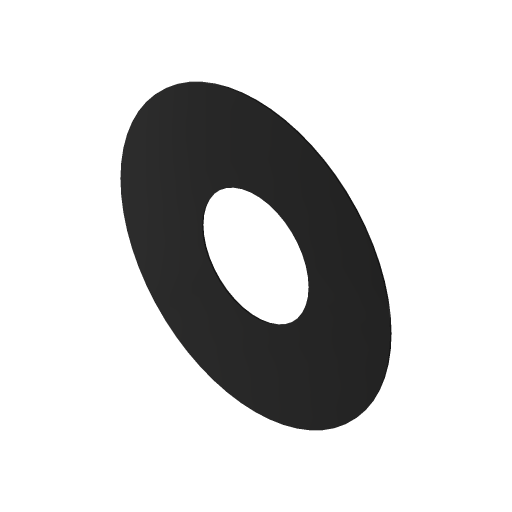
# Autodesk Inventor part: E-Stop Plate (Black)
Saved by Autodesk Inventor 2023.2 (Build 272271000, 271)
## iProperties
Created: 2021-03-05
Part Number: E-Stop Plate (Black)
Material: UHMW, Black
Document SubType Name: Modeling
Designer: Remo
Mass: 0.634081 g
Surface Area: 45.736 cm^2
Volume: 0.674554 cm^3
Density: 0.94 g/cm^3
Appearance: Smooth - Black
Author: Remo
Autodesk Inventor part; units mm, degrees
ref_plane "YZ Plane" through (0, 0, 0) normal (1, 0, 0) x (0, 1, 0)
ref_plane "XZ Plane" through (0, 0, 0) normal (0, 1, 0) x (-1, 0, 0)
ref_plane "XY Plane" through (0, 0, 0) normal (0, 0, 1) x (1, 0, 0)
sketch "Sketch1" plane through (0, 0, 0) normal (0, 0, 1) x (1, 0, 0)
  circle A0 centre (0, 0) radius 29.12 projected
  spline S0 degree 3 poles (-11.9075, -16.7717) (-12.086, -16.7855) (-12.2588, -16.8244) (-12.5934, -16.9566) (-12.7523, -17.0491) (-13.1401, -17.3576) (-13.3337, -17.6127) (-13.4879, -17.8856) knots -0.20259 -0.20259 -0.20259 -0.20259 -0.148567 -0.148567 -0.094046 -0.094046 0 0 0 0 projected
  spline S1 degree 3 poles (-10.0812, -17.2756) (-10.3794, -17.1072) (-10.7111, -16.9507) (-11.3404, -16.7781) (-11.626, -16.7509) (-11.9075, -16.7717) knots -0.178551 -0.178551 -0.178551 -0.178551 -0.084682 -0.084682 0 0 0 0 projected
  line L0 (-7.7154, -18.612) -> (-10.0812, -17.2756) projected
  line L1 (-11.1583, -24.7069) -> (-7.7154, -18.612) projected
  line L2 (-12.6894, -23.8419) -> (-11.1583, -24.7069) projected
  line L3 (-11.5622, -21.8466) -> (-12.6894, -23.8419) projected
  line L4 (-12.3624, -21.3946) -> (-11.5622, -21.8466) projected
  spline S2 degree 3 poles (-13.3296, -20.5811) (-13.2082, -20.736) (-13.0703, -20.8775) (-12.8431, -21.0755) (-12.6688, -21.2215) (-12.3624, -21.3946) knots -0.304465 -0.304465 -0.304465 -0.304465 -0.105593 -0.105593 0 0 0 0 projected
  spline S3 degree 3 poles (-13.7846, -19.6335) (-13.7433, -19.8022) (-13.685, -19.9651) (-13.5697, -20.2108) (-13.4849, -20.3798) (-13.3296, -20.5811) knots -0.211773 -0.211773 -0.211773 -0.211773 -0.07625 -0.07625 0 0 0 0 projected
  spline S4 degree 3 poles (-13.4879, -17.8856) (-13.5813, -18.0509) (-13.6584, -18.2235) (-13.7744, -18.5785) (-13.8153, -18.7636) (-13.8576, -19.177) (-13.845, -19.408) (-13.7846, -19.6335) knots -0.181189 -0.181189 -0.181189 -0.181189 -0.12469 -0.12469 -0.070002 -0.070002 0 0 0 0 projected
  spline S5 degree 3 poles (-3.098, -19.6093) (-3.5995, -19.53) (-4.1119, -19.5258) (-4.9872, -19.7428) (-5.336, -19.9081) (-5.8954, -20.327) (-6.2031, -20.6109) (-6.7632, -21.5612) (-6.9293, -22.1193) (-7.0183, -22.6822) knots -0.803042 -0.803042 -0.803042 -0.803042 -0.536977 -0.536977 -0.330685 -0.330685 -0.170955 -0.170955 0 0 0 0 projected
  spline S6 degree 3 poles (-0.3227, -23.741) (-0.2718, -23.4189) (-0.2455, -23.0908) (-0.2648, -22.4708) (-0.3034, -22.1789) (-0.5023, -21.4398) (-0.6961, -21.0977) (-1.1107, -20.5353) (-1.3922, -20.2811) (-2.1435, -19.8313) (-2.6154, -19.6856) (-3.098, -19.6093) knots -0.479254 -0.479254 -0.479254 -0.479254 -0.41452 -0.41452 -0.356105 -0.356105 -0.262594 -0.262594 -0.146589 -0.146589 0 0 0 0 projected
  spline S7 degree 3 poles (-4.2374, -26.8147) (-3.7386, -26.8936) (-3.2285, -26.8982) (-2.3601, -26.6833) (-2.015, -26.5203) (-1.4323, -26.0851) (-1.1292, -25.7911) (-0.5788, -24.861) (-0.4118, -24.3043) (-0.3227, -23.741) knots -0.728851 -0.728851 -0.728851 -0.728851 -0.500216 -0.500216 -0.324019 -0.324019 -0.171091 -0.171091 0 0 0 0 projected
  spline S8 degree 3 poles (-7.0183, -22.6822) (-7.0686, -23.0001) (-7.0951, -23.3241) (-7.079, -23.9356) (-7.043, -24.2235) (-6.8418, -24.9989) (-6.6342, -25.3416) (-6.2365, -25.8816) (-5.9526, -26.1383) (-5.1963, -26.5915) (-4.7225, -26.738) (-4.2374, -26.8147) knots -0.448983 -0.448983 -0.448983 -0.448983 -0.396063 -0.396063 -0.348437 -0.348437 -0.26439 -0.26439 -0.147326 -0.147326 0 0 0 0 projected
  spline S9 degree 3 poles (9.7964, -22.9748) (9.873, -23.1091) (9.9611, -23.2363) (10.1586, -23.4637) (10.2652, -23.5632) (10.5993, -23.8097) (10.8409, -23.9174) (11.3557, -24.0436) (11.7011, -24.0855) (12.6436, -23.9411) (13.1336, -23.7358) (13.5793, -23.4816) knots -0.573293 -0.573293 -0.573293 -0.573293 -0.495269 -0.495269 -0.421354 -0.421354 -0.285769 -0.285769 -0.153911 -0.153911 0 0 0 0 projected
  spline S10 degree 3 poles (10.1128, -20.6327) (9.9812, -20.7887) (9.8593, -20.9571) (9.6734, -21.2903) (9.6029, -21.4546) (9.5083, -21.8196) (9.4931, -22.0143) (9.5618, -22.4912) (9.6645, -22.7435) (9.7964, -22.9748) knots -0.267973 -0.267973 -0.267973 -0.267973 -0.2019 -0.2019 -0.14446 -0.14446 -0.079889 -0.079889 0 0 0 0 projected
  spline S11 degree 3 poles (11.1303, -19.6344) (10.9594, -19.7906) (10.7883, -19.9482) (10.4605, -20.2529) (10.3598, -20.3495) (10.1128, -20.6327) knots -0.233565 -0.233565 -0.233565 -0.233565 -0.112749 -0.112749 0 0 0 0 projected
  spline S12 degree 3 poles (11.5822, -18.5604) (11.612, -18.6128) (11.6358, -18.6685) (11.6628, -18.7815) (11.667, -18.8365) (11.6526, -18.9826) (11.6201, -19.0532) (11.5167, -19.2467) (11.3517, -19.4308) (11.1303, -19.6344) knots -0.147436 -0.147436 -0.147436 -0.147436 -0.130795 -0.130795 -0.115368 -0.115368 -0.09026 -0.09026 0 0 0 0 projected
  spline S13 degree 3 poles (10.9597, -18.282) (11.0119, -18.2769) (11.064, -18.2773) (11.169, -18.2893) (11.2208, -18.301) (11.3587, -18.3464) (11.4141, -18.3806) (11.5054, -18.451) (11.5486, -18.5016) (11.5822, -18.5604) knots -0.050985 -0.050985 -0.050985 -0.050985 -0.042849 -0.042849 -0.034581 -0.034581 -0.020323 -0.020323 0 0 0 0 projected
  spline S14 degree 3 poles (10.1862, -18.5403) (10.305, -18.4726) (10.4335, -18.4094) (10.6285, -18.342) (10.7569, -18.3024) (10.9597, -18.282) knots -0.181503 -0.181503 -0.181503 -0.181503 -0.061137 -0.061137 0 0 0 0 projected
  spline S15 degree 3 poles (8.7516, -20.2728) (8.8988, -19.8634) (9.1304, -19.5268) (9.5456, -18.9963) (9.8398, -18.7379) (10.1862, -18.5403) knots -0.202104 -0.202104 -0.202104 -0.202104 -0.119641 -0.119641 0 0 0 0 projected
  line L5 (8.6186, -20.3487) -> (8.7516, -20.2728) projected
  line L6 (7.826, -18.9592) -> (8.6186, -20.3487) projected
  spline S16 degree 3 poles (9.6327, -17.3866) (9.2693, -17.594) (8.9309, -17.8365) (8.3425, -18.3546) (8.0628, -18.6388) (7.826, -18.9592) knots -0.256315 -0.256315 -0.256315 -0.256315 -0.119514 -0.119514 0 0 0 0 projected
  spline S17 degree 3 poles (13.251, -17.8567) (13.1848, -17.7407) (13.1089, -17.631) (12.9386, -17.4329) (12.8465, -17.3454) (12.5438, -17.1152) (12.3176, -17.0112) (11.7887, -16.8735) (11.4213, -16.8389) (10.5222, -16.9611) (10.0601, -17.1429) (9.6327, -17.3866) knots -0.489668 -0.489668 -0.489668 -0.489668 -0.433118 -0.433118 -0.379048 -0.379048 -0.272086 -0.272086 -0.147592 -0.147592 0 0 0 0 projected
  spline S18 degree 3 poles (12.9162, -20.3268) (13.0547, -20.1676) (13.1845, -19.9949) (13.3806, -19.6559) (13.4552, -19.4893) (13.5341, -19.1934) (13.5804, -18.9652) (13.5005, -18.3783) (13.3939, -18.1073) (13.251, -17.8567) knots -0.461771 -0.461771 -0.461771 -0.461771 -0.308608 -0.308608 -0.177631 -0.177631 -0.086532 -0.086532 0 0 0 0 projected
  spline S19 degree 3 poles (11.7818, -21.4179) (11.9665, -21.2344) (12.1601, -21.056) (12.4294, -20.8205) (12.663, -20.6175) (12.9162, -20.3268) knots -0.424502 -0.424502 -0.424502 -0.424502 -0.115659 -0.115659 0 0 0 0 projected
  spline S20 degree 3 poles (11.5074, -22.345) (11.4826, -22.3016) (11.4628, -22.2558) (11.4371, -22.1618) (11.431, -22.1152) (11.4331, -21.9724) (11.4615, -21.8956) (11.5529, -21.6815) (11.6558, -21.5407) (11.7818, -21.4179) knots -0.087282 -0.087282 -0.087282 -0.087282 -0.078342 -0.078342 -0.069852 -0.069852 -0.052789 -0.052789 0 0 0 0 projected
  spline S21 degree 3 poles (12.1847, -22.6509) (12.1253, -22.6572) (12.0659, -22.658) (11.948, -22.6472) (11.8906, -22.636) (11.7833, -22.6034) (11.7243, -22.5804) (11.5982, -22.4806) (11.5477, -22.4157) (11.5074, -22.345) knots -0.101132 -0.101132 -0.101132 -0.101132 -0.074483 -0.074483 -0.048246 -0.048246 -0.024412 -0.024412 0 0 0 0 projected
  spline S22 degree 3 poles (12.942, -22.3757) (12.8032, -22.4549) (12.6097, -22.5333) (12.4074, -22.6084) (12.2905, -22.6418) (12.1847, -22.6509) knots -0.057311 -0.057311 -0.057311 -0.057311 -0.031864 -0.031864 0 0 0 0 projected
  spline S23 degree 3 poles (14.5555, -20.3844) (14.3497, -20.9514) (14.0707, -21.3431) (13.5958, -21.9066) (13.2936, -22.1752) (12.942, -22.3757) knots -0.221118 -0.221118 -0.221118 -0.221118 -0.12144 -0.12144 0 0 0 0 projected
  line L7 (14.6935, -20.3057) -> (14.5555, -20.3844) projected
  line L8 (15.5198, -21.7544) -> (14.6935, -20.3057) projected
  spline S24 degree 3 poles (13.5793, -23.4816) (13.9855, -23.2499) (14.3927, -22.9722) (14.8147, -22.5631) (15.1635, -22.2305) (15.5198, -21.7544) knots -0.877949 -0.877949 -0.877949 -0.877949 -0.178404 -0.178404 0 0 0 0 projected
  spline S25 degree 3 poles (-18.1304, 8.8173) (-17.9728, 8.9559) (-17.818, 9.1055) (-17.6216, 9.3271) (-17.4778, 9.4935) (-17.2255, 9.9064) knots -0.498689 -0.498689 -0.498689 -0.498689 -0.145143 -0.145143 0 0 0 0 projected
  spline S26 degree 3 poles (-18.9751, 8.1967) (-18.8415, 8.2847) (-18.7005, 8.3801) (-18.4363, 8.5607) (-18.3335, 8.6325) (-18.1304, 8.8173) knots -0.1644 -0.1644 -0.1644 -0.1644 -0.08237 -0.08237 0 0 0 0 projected
  line L9 (-20.3788, 9.0546) -> (-18.9751, 8.1967) projected
  line L10 (-20.2959, 9.1902) -> (-20.3788, 9.0546) projected
  spline S27 degree 3 poles (-19.4381, 9.5168) (-19.5873, 9.4382) (-19.7448, 9.3669) (-20.0344, 9.2701) (-20.1646, 9.2282) (-20.2959, 9.1902) knots -0.091625 -0.091625 -0.091625 -0.091625 -0.04101 -0.04101 0 0 0 0 projected
  spline S28 degree 3 poles (-18.4974, 10.338) (-18.6159, 10.1442) (-18.763, 9.9756) (-19.0246, 9.769) (-19.221, 9.6191) (-19.4381, 9.5168) knots -0.226077 -0.226077 -0.226077 -0.226077 -0.071989 -0.071989 0 0 0 0 projected
  spline S29 degree 3 poles (-18.2577, 11.6874) (-18.2301, 11.5674) (-18.2142, 11.4455) (-18.2108, 11.2035) (-18.2223, 11.0859) (-18.271, 10.8619) (-18.3291, 10.6134) (-18.4974, 10.338) knots -0.30907 -0.30907 -0.30907 -0.30907 -0.201049 -0.201049 -0.096825 -0.096825 0 0 0 0 projected
  spline S30 degree 3 poles (-19.4782, 13.1713) (-19.2716, 13.045) (-19.0679, 12.8996) (-18.8111, 12.6601) (-18.6531, 12.5037) (-18.3913, 12.0891) (-18.3034, 11.895) (-18.2577, 11.6874) knots -0.332846 -0.332846 -0.332846 -0.332846 -0.14713 -0.14713 -0.063762 -0.063762 0 0 0 0 projected
  spline S31 degree 3 poles (-21.3232, 13.6008) (-21.1949, 13.6303) (-21.0629, 13.6415) (-20.7812, 13.6376) (-20.6299, 13.6185) (-20.3205, 13.5566) (-19.9732, 13.4738) (-19.4782, 13.1713) knots -0.470219 -0.470219 -0.470219 -0.470219 -0.331835 -0.331835 -0.174011 -0.174011 0 0 0 0 projected
  spline S32 degree 3 poles (-22.4604, 12.7735) (-22.3904, 12.8881) (-22.3109, 12.9967) (-22.1518, 13.1717) (-22.0549, 13.2662) (-21.7548, 13.4737) (-21.5411, 13.5527) (-21.3232, 13.6008) knots -0.165131 -0.165131 -0.165131 -0.165131 -0.109374 -0.109374 -0.066951 -0.066951 0 0 0 0 projected
  spline S33 degree 3 poles (-22.7512, 11.6016) (-22.7536, 11.8007) (-22.7322, 11.9986) (-22.6728, 12.2859) (-22.6229, 12.5076) (-22.4604, 12.7735) knots -0.290938 -0.290938 -0.290938 -0.290938 -0.093474 -0.093474 0 0 0 0 projected
  spline S34 degree 3 poles (-22.6539, 10.6513) (-22.6764, 10.7846) (-22.6988, 10.9358) (-22.7398, 11.2265) (-22.7525, 11.3258) (-22.7512, 11.6016) knots -0.152838 -0.152838 -0.152838 -0.152838 -0.082731 -0.082731 0 0 0 0 projected
  line L11 (-22.7456, 10.5012) -> (-22.6539, 10.6513) projected
  line L12 (-24.1686, 11.3709) -> (-22.7456, 10.5012) projected
  spline S35 degree 3 poles (-24.0083, 12.4164) (-24.0532, 12.2392) (-24.0867, 12.0524) (-24.1234, 11.7895) (-24.1547, 11.5642) (-24.1686, 11.3709) knots -0.18646 -0.18646 -0.18646 -0.18646 -0.058134 -0.058134 0 0 0 0 projected
  spline S36 degree 3 poles (-23.4336, 13.694) (-23.5626, 13.4829) (-23.6852, 13.2575) (-23.818, 12.9482) (-23.9164, 12.7188) (-24.0083, 12.4164) knots -0.358594 -0.358594 -0.358594 -0.358594 -0.094817 -0.094817 0 0 0 0 projected
  spline S37 degree 3 poles (-18.5364, 14.7231) (-18.7987, 14.8834) (-19.0745, 15.0241) (-19.6236, 15.2337) (-19.8939, 15.3075) (-20.7042, 15.4239) (-21.1195, 15.3562) (-21.7799, 15.196) (-22.1388, 15.0282) (-22.8594, 14.4946) (-23.1768, 14.114) (-23.4336, 13.694) knots -0.441637 -0.441637 -0.441637 -0.441637 -0.394486 -0.394486 -0.351486 -0.351486 -0.26892 -0.26892 -0.147692 -0.147692 0 0 0 0 projected
  spline S38 degree 3 poles (-17.2255, 9.9064) (-17.0775, 10.1485) (-16.9489, 10.4033) (-16.7596, 10.9132) (-16.6948, 11.1645) (-16.606, 11.8736) (-16.6598, 12.2507) (-16.8368, 12.9354) (-17.0169, 13.2931) (-17.6046, 14.0668) (-18.0556, 14.4292) (-18.5364, 14.7231) knots -0.488562 -0.488562 -0.488562 -0.488562 -0.432469 -0.432469 -0.381055 -0.381055 -0.291208 -0.291208 -0.169067 -0.169067 0 0 0 0 projected
  line L13 (-9.1859, 17.9401) -> (-4.7403, 19.5582) projected
  line L14 (-9.6419, 19.1928) -> (-9.1859, 17.9401) projected
  line L15 (-6.838, 20.2133) -> (-9.6419, 19.1928) projected
  line L16 (-7.4434, 21.8764) -> (-6.838, 20.2133) projected
  line L17 (-10.0287, 20.9355) -> (-7.4434, 21.8764) projected
  line L18 (-10.4846, 22.1881) -> (-10.0287, 20.9355) projected
  line L19 (-7.8993, 23.1291) -> (-10.4846, 22.1881) projected
  line L20 (-8.3203, 24.2858) -> (-7.8993, 23.1291) projected
  line L21 (-11.1242, 23.2653) -> (-8.3203, 24.2858) projected
  line L22 (-11.5801, 24.518) -> (-11.1242, 23.2653) projected
  line L23 (-7.1345, 26.1361) -> (-11.5801, 24.518) projected
  line L24 (-4.7403, 19.5582) -> (-7.1345, 26.1361) projected
  line L25 (10.0397, 17.4767) -> (13.8185, 14.6302) projected
  line L26 (10.8417, 18.5415) -> (10.0397, 17.4767) projected
  line L27 (13.225, 16.7462) -> (10.8417, 18.5415) projected
  line L28 (14.2899, 18.1599) -> (13.225, 16.7462) projected
  line L29 (12.0924, 19.8152) -> (14.2899, 18.1599) projected
  line L30 (12.8944, 20.88) -> (12.0924, 19.8152) projected
  line L31 (15.092, 19.2247) -> (12.8944, 20.88) projected
  line L32 (15.8326, 20.2079) -> (15.092, 19.2247) projected
  line L33 (13.4493, 22.0031) -> (15.8326, 20.2079) projected
  line L34 (14.2513, 23.0679) -> (13.4493, 22.0031) projected
  line L35 (18.0302, 20.2215) -> (14.2513, 23.0679) projected
  line L36 (13.8185, 14.6302) -> (18.0302, 20.2215) projected
  line L37 (19.0555, 6.5665) -> (20.031, 1.9372) projected
  line L38 (20.3599, 6.8414) -> (19.0555, 6.5665) projected
  line L39 (20.9752, 3.9217) -> (20.3599, 6.8414) projected
  line L40 (22.707, 4.2867) -> (20.9752, 3.9217) projected
  line L41 (22.1397, 6.9788) -> (22.707, 4.2867) projected
  line L42 (23.4441, 7.2537) -> (22.1397, 6.9788) projected
  line L43 (24.0114, 4.5616) -> (23.4441, 7.2537) projected
  line L44 (25.2159, 4.8154) -> (24.0114, 4.5616) projected
  line L45 (24.6006, 7.7351) -> (25.2159, 4.8154) projected
  line L46 (25.905, 8.01) -> (24.6006, 7.7351) projected
  line L47 (26.8806, 3.3807) -> (25.905, 8.01) projected
  line L48 (20.031, 1.9372) -> (26.8806, 3.3807) projected
  line L49 (20.865, 17.505) -> (14.9583, 13.7484) projected
  line L50 (21.9518, 15.7961) -> (20.865, 17.505) projected
  line L51 (19.8647, 12.6403) -> (21.9518, 15.7961) projected
  line L52 (23.6139, 13.1827) -> (19.8647, 12.6403) projected
  line L53 (24.7007, 11.4738) -> (23.6139, 13.1827) projected
  line L54 (18.794, 7.7173) -> (24.7007, 11.4738) projected
  line L55 (17.9051, 9.115) -> (18.794, 7.7173) projected
  line L56 (21.8205, 11.6052) -> (17.9051, 9.115) projected
  line L57 (18.6113, 11.07) -> (21.8205, 11.6052) projected
  line L58 (17.966, 12.0848) -> (18.6113, 11.07) projected
  line L59 (19.8114, 14.7643) -> (17.966, 12.0848) projected
  line L60 (15.8959, 12.2742) -> (19.8114, 14.7643) projected
  line L61 (14.9583, 13.7484) -> (15.8959, 12.2742) projected
  line L62 (6.077, 22.2007) -> (2.8939, 20.1322) projected
  spline S39 degree 3 poles (5.4854, 24.6157) (5.3939, 24.3447) (5.334, 24.0582) (5.338, 23.5934) (5.3641, 23.3518) (5.6291, 22.7239) (5.8294, 22.4447) (6.077, 22.2007) knots -0.364955 -0.364955 -0.364955 -0.364955 -0.204435 -0.204435 -0.104304 -0.104304 0 0 0 0 projected
  spline S40 degree 3 poles (6.7548, 25.8217) (6.5791, 25.7785) (6.4123, 25.7125) (6.0098, 25.4761) (5.8713, 25.315) (5.6751, 25.0793) (5.5644, 24.8496) (5.4854, 24.6157) knots -0.103229 -0.103229 -0.103229 -0.103229 -0.09192 -0.09192 -0.074055 -0.074055 0 0 0 0 projected
  spline S41 degree 3 poles (8.5944, 25.5957) (8.2806, 25.7016) (7.9367, 25.799) (7.4715, 25.8723) (7.1572, 25.9142) (6.7548, 25.8217) knots -0.419777 -0.419777 -0.419777 -0.419777 -0.123883 -0.123883 0 0 0 0 projected
  line L63 (11.2602, 24.6956) -> (8.5944, 25.5957) projected
  line L64 (9.0208, 18.0634) -> (11.2602, 24.6956) projected
  line L65 (7.3655, 18.6224) -> (9.0208, 18.0634) projected
  line L66 (8.1875, 21.057) -> (7.3655, 18.6224) projected
  line L67 (7.5856, 21.2603) -> (8.1875, 21.057) projected
  line L68 (4.9201, 19.448) -> (7.5856, 21.2603) projected
  line L69 (2.8939, 20.1322) -> (4.9201, 19.448) projected
  line L70 (-3.5721, 23.765) -> (-3.4869, 20.3171) projected
  line L71 (-0.5155, 23.8406) -> (-3.5721, 23.765) projected
  line L72 (-0.4832, 22.5306) -> (-0.5155, 23.8406) projected
  line L73 (-1.8385, 22.4971) -> (-0.4832, 22.5306) projected
  line L74 (-1.8044, 21.1191) -> (-1.8385, 22.4971) projected
  spline S42 degree 3 poles (-1.3617, 21.113) (-1.434, 21.1112) (-1.5108, 21.1117) (-1.6314, 21.1142) (-1.7172, 21.1161) (-1.8044, 21.1191) knots -0.065191 -0.065191 -0.065191 -0.065191 -0.026183 -0.026183 0 0 0 0 projected
  spline S43 degree 3 poles (0.8702, 23.5627) (0.8759, 23.3307) (0.8652, 23.0942) (0.7969, 22.6669) (0.7454, 22.471) (0.5802, 22.0866) (0.4638, 21.9055) (0.1991, 21.6361) (-0.0009, 21.4572) (-0.6536, 21.1791) (-1.0086, 21.1217) (-1.3617, 21.113) knots -0.647494 -0.647494 -0.647494 -0.647494 -0.49232 -0.49232 -0.358299 -0.358299 -0.212691 -0.212691 -0.105964 -0.105964 0 0 0 0 projected
  spline S44 degree 3 poles (0.2265, 25.2718) (0.3242, 25.1769) (0.4092, 25.0712) (0.563, 24.8335) (0.629, 24.7017) (0.7463, 24.4093) (0.8571, 24.0909) (0.8702, 23.5627) knots -0.425401 -0.425401 -0.425401 -0.425401 -0.297011 -0.297011 -0.158513 -0.158513 0 0 0 0 projected
  spline S45 degree 3 poles (-1.2678, 25.808) (-0.8998, 25.8171) (-0.6167, 25.7527) (-0.165, 25.5802) (0.0435, 25.446) (0.2265, 25.2718) knots -0.145071 -0.145071 -0.145071 -0.145071 -0.075784 -0.075784 0 0 0 0 projected
  spline S46 degree 3 poles (-2.597, 25.4063) (-2.4106, 25.522) (-2.2044, 25.6118) (-1.8895, 25.7185) (-1.6371, 25.7989) (-1.2678, 25.808) knots -0.325583 -0.325583 -0.325583 -0.325583 -0.110815 -0.110815 0 0 0 0 projected
  spline S47 degree 3 poles (-3.4104, 24.7961) (-3.3055, 24.8814) (-3.1562, 25.0028) (-2.9957, 25.1335) (-2.8208, 25.2759) (-2.597, 25.4063) knots -0.212632 -0.212632 -0.212632 -0.212632 -0.077698 -0.077698 0 0 0 0 projected
  line L75 (-3.5692, 24.7921) -> (-3.4104, 24.7961) projected
  line L76 (-3.6098, 26.4367) -> (-3.5692, 24.7921) projected
  spline S48 degree 3 poles (-1.0619, 27.1182) (-1.5619, 27.1058) (-2.0723, 27.0529) (-2.8731, 26.7876) (-3.2482, 26.6234) (-3.6098, 26.4367) knots -0.253073 -0.253073 -0.253073 -0.253073 -0.122087 -0.122087 0 0 0 0 projected
  spline S49 degree 3 poles (2.6856, 23.5792) (2.6782, 23.877) (2.6468, 24.1748) (2.525, 24.7335) (2.44, 24.9934) (2.1131, 25.688) (1.8437, 26.0041) (1.2967, 26.5156) (0.9432, 26.7311) (0.0351, 27.0685) (-0.5156, 27.1317) (-1.0619, 27.1182) knots -0.502065 -0.502065 -0.502065 -0.502065 -0.442916 -0.442916 -0.388497 -0.388497 -0.290476 -0.290476 -0.163933 -0.163933 0 0 0 0 projected
  spline S50 degree 3 poles (-0.8308, 19.838) (-0.5152, 19.8458) (-0.199, 19.8798) (0.39, 20.0131) (0.6621, 20.106) (1.3491, 20.4478) (1.6399, 20.7085) (2.1074, 21.215) (2.3102, 21.5578) (2.6393, 22.4602) (2.6993, 23.0248) (2.6856, 23.5792) knots -0.480218 -0.480218 -0.480218 -0.480218 -0.424147 -0.424147 -0.372991 -0.372991 -0.287915 -0.287915 -0.166369 -0.166369 0 0 0 0 projected
  spline S51 degree 3 poles (-3.4869, 20.3171) (-3.1169, 20.1769) (-2.6681, 20.0643) (-2.0696, 19.9343) (-1.5259, 19.8209) (-0.8308, 19.838) knots -0.581904 -0.581904 -0.581904 -0.581904 -0.208577 -0.208577 0 0 0 0 projected
  line L77 (-19.3094, 19.1107) -> (-14.9108, 13.6654) projected
  line L78 (-18.0606, 20.1195) -> (-19.3094, 19.1107) projected
  line L79 (-15.5405, 16.9996) -> (-18.0606, 20.1195) projected
  line L80 (-16.322, 21.5239) -> (-15.5405, 16.9996) projected
  line L81 (-14.6451, 22.8784) -> (-16.322, 21.5239) projected
  line L82 (-10.2465, 17.4331) -> (-14.6451, 22.8784) projected
  line L83 (-11.4953, 16.4243) -> (-10.2465, 17.4331) projected
  line L84 (-14.5608, 20.2193) -> (-11.4953, 16.4243) projected
  line L85 (-13.5958, 14.7276) -> (-14.5608, 20.2193) projected
  line L86 (-14.9108, 13.6654) -> (-13.5958, 14.7276) projected
  line L87 (-26.6074, 4.7659) -> (-27.0402, 2.8748) projected
  line L88 (-23.8794, 5.4974) -> (-26.6074, 4.7659) projected
  line L89 (-26.0075, 7.3869) -> (-23.8794, 5.4974) projected
  line L90 (-25.5607, 9.3389) -> (-26.0075, 7.3869) projected
  line L91 (-22.05, 6.0156) -> (-25.5607, 9.3389) projected
  line L92 (-19.2852, 5.3828) -> (-22.05, 6.0156) projected
  line L93 (-19.6775, 3.6686) -> (-19.2852, 5.3828) projected
  line L94 (-22.5253, 4.3204) -> (-19.6775, 3.6686) projected
  line L95 (-27.0402, 2.8748) -> (-22.5253, 4.3204) projected
  line L96 (4.3092, -26.6684) -> (6.0352, -26.3315) projected
  line L97 (3.2236, -21.1064) -> (4.3092, -26.6684) projected
  line L98 (1.1915, -21.503) -> (3.2236, -21.1064) projected
  line L99 (0.9361, -20.1947) -> (1.1915, -21.503) projected
  line L100 (6.7264, -19.0645) -> (0.9361, -20.1947) projected
  line L101 (6.9817, -20.3729) -> (6.7264, -19.0645) projected
  line L102 (4.9496, -20.7696) -> (6.9817, -20.3729) projected
  line L103 (6.0352, -26.3315) -> (4.9496, -20.7696) projected
  circle A1 centre (0, 0) radius 11.5 projected
extrude "Extrusion1" add sketch "Sketch1" along normal blind 0.3 contours A0 | S1 L0 L1 L2 L3 L4 S2 S3 S4 S0 | S6 S7 S8 S5 | S10 S11 S12 S13 S14 S15 L5 L6 S16 S17 S18 S19 S20 S21 S22 S23 L7 L8 S24 S9 | S26 L9 L10 S27 S28 S29 S30 S31 S32 S33 S34 L11 L12 S35 S36 S37 S38 S25 | L14 L15 L16 L17 L18 L19 L20 L21 L22 L23 L24 L13 | L26 L27 L28 L29 L30 L31 L32 L33 L34 L35 L36 L25 | L38 L39 L40 L41 L42 L43 L44 L45 L46 L47 L48 L37 | L50 L51 L52 L53 L54 L55 L56 L57 L58 L59 L60 L61 L49 | S39 S40 S41 L63 L64 L65 L66 L67 L68 L69 L62 | L71 L72 L73 L74 S42 S43 S44 S45 S46 S47 L75 L76 S48 S49 S50 S51 L70 | L78 L79 L80 L81 L82 L83 L84 L85 L86 L77 | L88 L89 L90 L91 L92 L93 L94 L95 L87 | L97 L98 L99 L100 L101 L102 L103 L96
body "Solid1"
